IKEA Filamentstorage (Autodesk Fusion 360 design; units mm, degrees)
Autodesk Fusion 360 part; units mm, degrees
sketch "Sketch1" plane through (0, 0, 0) normal (1, 0, 0) x (0, 1, 0)
  circle A0 centre (0, 0) radius 9
  dimension "d1" = 18
  constraint coincident A0.centre origin
  measures "d1" diameter of A0
extrude "Extrude1" add sketch "Sketch1" along normal blind 100 from surface at 5 contours A0 picked at (-5.167563, 0.326708) makes body 1
sketch "Sketch2" plane through (0, 0, 0) normal (1, 0, 0) x (0, 1, 0)
  circle A0 centre (0, 0) radius 9.2
  circle A1 centre (0, 0) radius 11.7
  line L0 (0, 0) -> (-19.923894, 1.743115)
  line L1 (0, 0) -> (20, 0) construction
  line L2 (0, 0) -> (19.923894, 1.743115)
  line L3 (0, 0) -> (20, 0) construction
  circle A2 centre (-12.792942, 10.734553) radius 5
  circle A3 centre (12.792942, 10.734553) radius 5
  circle A4 centre (0, -16.7) radius 5
  line L4 (0, 0) -> (-14.625231, 12.272026)
  line L5 (0, 0) -> (29.154759, 0) construction
  line L6 (0, 0) -> (14.78669, 12.407507)
  line L7 (0, 0) -> (37.611272, 0) construction
  line L8 (-18.989323, 11.979964) -> (-9.922984, -6.326611)
  line L9 (9.445604, -7.290526) -> (18.396944, 10.783844)
  line L10 (-15.030342, 15.734553) -> (16.223429, 15.734553)
  line L11 (4.061867, -19.888862) -> (12.280307, -1.124988)
  line L12 (-12.660272, -0.257474) -> (-3.606521, -20.928484)
  circle A5 centre (-12.792942, 10.734553) radius 1.5
  circle A6 centre (12.792942, 10.734553) radius 1.5
  circle A7 centre (0, -16.7) radius 1.5
  dimension "d4" = 18.4
  dimension "d5" = 23.4
  dimension "d8" = 175
  dimension "d9" = 20
  dimension "d10" = 20
  dimension "d11" = 5
  dimension "d39" = 10
  dimension "d40" = 10
  dimension "d41" = 10
  dimension "d42" = 140
  dimension "d44" = 40
  dimension "d45" = 3
  dimension "d46" = 3
  dimension "d47" = 3
  constraint coincident A0.centre A1.centre
  constraint horizontal L1
  constraint horizontal L3
  constraint vertical A0.centre A4.centre
  constraint tangent A1 A4
  constraint horizontal L5
  constraint tangent A1 A2
  constraint tangent A1 A3
  constraint horizontal L7
  constraint tangent A2 L8
  constraint tangent A3 L9
  constraint tangent A2 L10
  constraint tangent A3 L10
  constraint tangent A1 L8
  constraint tangent A1 L9
  constraint tangent A1 L11
  constraint tangent A4 L11
  constraint tangent A4 L12
  constraint tangent A1 L12
  constraint concentric A2 A5
  constraint concentric A3 A6
  constraint concentric A4 A7
  measures "d4" diameter of A0
  measures "d5" diameter of A1
  measures "d8" angle of L0 L1
  measures "d11" angle of L2 L3
  measures "d39" diameter of A2
  measures "d40" diameter of A3
  measures "d41" diameter of A4
  measures "d42" angle of L4 L5
  measures "d44" angle of L6 L7
  measures "d45" diameter of A5
  measures "d46" diameter of A6
  measures "d47" diameter of A7
extrude "Extrude2" add sketch "Sketch2" along normal blind 2 separate body contours A0 L0 L2 | A0 A1 L0 L2 | A0 L2 L6 | A0 A1 L2 L6 | A0 A1 L0 L4 | A0 L0 L4 | A0 L4 L6 | A0 A1 L4 L6 | A1 L2 L9 L11 | A1 L2 A3 L9 | A1 L0 A2 L8 | A1 L0 L8 L12 | A1 A2 A3 L10 | A3 | A2 | A1 L8 L12 | A1 L9 L11 | A1 A4 L9 L11 | A1 A4 L8 L12 | A4 | L4 A5 | L4 A5 | L6 A6 | L6 A6 | A7 picked at (6.100364, -0.448469) picked at (-5.061649, -9.594578) picked at (5.899243, 1.636005) picked at (8.830312, 6.30119) picked at (-8.830312, 6.30119) picked at (-6.05465, 0.904873) picked at (-4.38791, 4.262092) picked at (-7.92948, 7.391485) picked at (12.312324, -0.136976) picked at (12.826387, 3.132192) picked at (-12.826387, 3.132192) picked at (-12.331571, 0.590696) picked at (0.006259, 13.58093) picked at (13.092305, 14.547042) picked at (-16.341094, 9.307831) picked at (-10.604561, -4.944988) picked at (10.604561, -4.944988) picked at (5.03693, -11.545648) picked at (-5.029871, -11.534757) picked at (0.277768, -20.514506) picked at (-12.78295, 10.184937) picked at (-12.370024, 11.297831) picked at (12.270917, 10.95906) picked at (13.247175, 10.525573) picked at (-0.349897, -17.261985) makes body 2
extrude "Extrude7" cut sketch "Sketch2" along normal blind 23 contours L4 A5 | L4 A5 | L6 A6 | L6 A6 | A7 picked at (-12.78295, 10.184937) picked at (-12.370024, 11.297831) picked at (12.270917, 10.95906) picked at (13.247175, 10.525573) picked at (-0.349897, -17.261985) bodies 2
copy_body "CopyPasteBodies1" bodies 2 makes body 3
move_body "Move2" bodies 3 to x (1, 0, 0) y (0, 1, 0) z (0, 0, 1) at (0, 75, 0)
extrude "Extrude3" add sketch "Sketch2" along normal blind 13 contours A0 A1 L0 L2 picked at (-5.061649, -9.594578) bodies 2
fillet "Fillet1" radius 2.5 1 edges at (2, 0, -11.7) on bodies 2
fillet "Fillet2" radius 0.75 4 edges at (7.5, 11.655478, 1.019722) (7.5, 9.164991, 0.801833) (7.5, -9.164991, 0.801833) (7.5, -11.655478, 1.019722) on bodies 2
sketch "Sketch3" plane through (0, 0, 0) normal (1, 0, 0) x (0, 1, 0)
  circle A0 centre (122.000002, 0) radius 9.2
  circle A1 centre (122.000002, 0) radius 12.2
  dimension "d54" = 18.4
  dimension "d55" = 24.4
  constraint concentric A0 A1
  measures "d54" diameter of A0
  measures "d55" diameter of A1
extrude "Extrude8" add sketch "Sketch3" along normal blind 8 separate body contours A1 picked at (133.120328, -1.063168) makes body 4
copy_body "CopyPasteBodies2" bodies 3 makes body 5
move_body "Move3" bodies 5 to x (1, 0, 0) y (0, 1, 0) z (0, 0, 1) at (0, 0, 200)
sketch "Sketch4" plane through (0, 0, 0) normal (-1, 0, 0) x (0, -1, 0)
  circle A0 centre (-62.207058, 210.734553) radius 1.5
  circle A1 centre (-87.792942, 210.734553) radius 1.5
  circle A2 centre (-75, 183.3) radius 1.5
  arc A3 (-57.726445, 208.51552) -> (-62.207058, 215.734553) centre (-62.207058, 210.734553) ccw
  line L0 (-62.207058, 215.734553) -> (-87.792942, 215.734553)
  arc A4 (-87.792942, 215.734553) -> (-92.273575, 208.515561) centre (-87.792942, 210.734553) ccw
  line L1 (-92.273575, 208.515561) -> (-85.606732, 195.054)
  line L2 (-85.606732, 195.054) -> (-79.579948, 181.293991)
  arc A5 (-79.579948, 181.293991) -> (-70.420042, 181.294012) centre (-75, 183.3) ccw
  line L3 (-70.420042, 181.294012) -> (-64.393268, 195.054)
  line L4 (-64.393268, 195.054) -> (-57.726445, 208.51552)
  line L5 (-100.035197, 285.734553) -> (-75.035197, 285.734553)
  line L6 (-75.035197, 285.734553) -> (-75.035197, 192.709018)
  line L7 (-75.035197, 192.709018) -> (-100.035197, 192.709018)
  line L8 (-100.035197, 192.709018) -> (-100.035197, 285.734553)
  dimension "d58" = 70
  dimension "d59" = 25
  constraint horizontal L5
  constraint vertical L6
  constraint horizontal L7
  constraint vertical L8
  measures "d58" distance of L0 L5
  measures "d59" distance of L6 L8
extrude "Extrude9" add sketch "Sketch4" along normal blind 0.4 separate body contours L0 A4 L1 L2 L5 L6 L7 L8 picked at (-87.621112, 262.40122) makes body 6
sketch "Sketch5" plane through (0, 0, 0) normal (1, 0, 0) x (0, 1, 0)
  line L0 (84.579647, 192.709018) -> (100.035197, 192.709018)
  line L1 (100.035197, 192.709018) -> (100.035197, 285.734553)
  line L2 (100.035197, 285.734553) -> (75.035197, 285.734553)
  line L3 (75.035197, 285.734553) -> (75.035197, 215.734553)
  line L4 (75.035197, 215.734553) -> (87.792942, 215.734553)
  arc A0 (92.273575, 208.515561) -> (87.792942, 215.734553) centre (87.792942, 210.734553) ccw
  line L5 (92.273575, 208.515561) -> (85.606732, 195.054)
  line L6 (85.606732, 195.054) -> (84.579647, 192.709018)
  line L7 (100.035197, 285.734553) -> (95.035197, 285.734553)
  line L8 (95.035197, 285.734553) -> (95.035197, 302.824671)
  line L9 (95.035197, 302.824671) -> (100.035197, 302.824671)
  line L10 (100.035197, 302.824671) -> (100.035197, 285.734553)
  dimension "d62" = 5
  constraint horizontal L7
  constraint vertical L8
  constraint horizontal L9
  constraint vertical L10
hidden bodies 1 5
